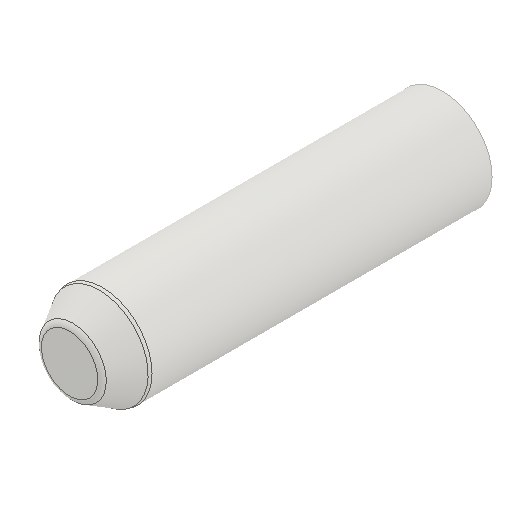
# Autodesk Inventor part: Testador Controle Remoto
Saved by Autodesk Inventor 2026.1 (Build 301233020, 233B)
## iProperties
Company: Elgin
Created: 2025-09-30
Material: Aço SAE 1045
Document SubType Name: Modeling
Designer: Willian Pinheiro
Mass: 89.1246 g
Surface Area: 35.9352 cm^2
Volume: 11.3535 cm^3
Density: 7.85 g/cm^3
Appearance: Aço
Description: Ponta Cilindro v1.1
Dimensões: Ø16 x 60 mm
Total: 1
Author: Willian Pinheiro
Title: Testador Controle Remoto
Revision Number: 01
Autodesk Inventor part; units mm, degrees
ref_plane "YZ Plane" through (0, 0, 0) normal (1, 0, 0) x (0, 1, 0)
ref_plane "XZ Plane" through (0, 0, 0) normal (0, 1, 0) x (-1, 0, 0)
ref_plane "XY Plane" through (0, 0, 0) normal (0, 0, 1) x (1, 0, 0)
sketch "Esboço1" plane through (0, 0, 0) normal (1, 0, 0) x (0, 1, 0)
  line L0 (-1.6, 0) -> (9.6, 0) construction
  line L1 (0, -42) -> (0, 42) construction
  line L2 (8, 30) -> (0, 30)
  line L3 (0, 30) -> (0, -30)
  line L4 (0, -30) -> (8, -30)
  line L5 (8, -30) -> (8, 30)
  line L6 (5.1132, 30) -> (8, 25)
  point P0 (0, 0)
  dimension "d0" = 16
  dimension "d1" = 60
  dimension "d2" = 5
  dimension "d3" = 30
  constraints: 10 end point, 3 point on line, 2 parallel, 1 horizontal, 1 perpendicular, 1 other
  measures "d0" diameter of L5 L3
  measures "d1" distance of L4.end L2.start
  measures "d2" vertical distance of L6.start L6.end
  measures "d3" angle of L5 L6
revolve "Revolução1" add sketch "Esboço1" angle 360 about axis through (0, 0, 30) along (0, 0, -1) contours L6 L5 L4 L3 L2
fillet "Arredondamento1" radius 1 2 edges at (0, -5.1132, 30) (0, -8, 25)
sketch "Esboço2" plane through (0, 0, -30) normal (0, 0, -1) x (-1, 0, 0)
  circle A0 centre (0, 0) radius 8 projected
  constraints: 1 coincident
hole "Furo1" at (0, 0, -30) direction (0, 0, 1) diameter 4.917 depth 20 tip angle 118 thread size "M6x1" class "6H" standard "ISO Metric profile"
